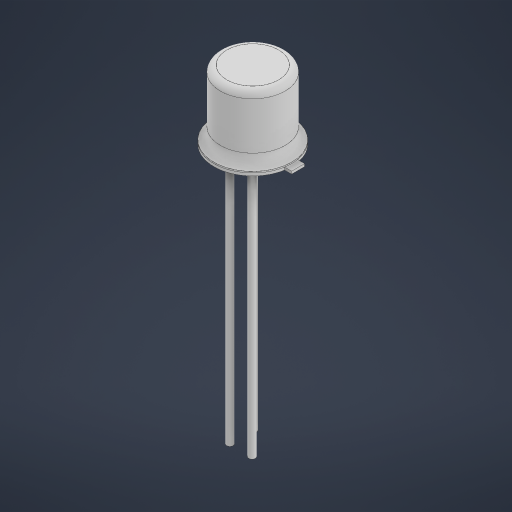
# Autodesk Inventor part: Part4
Saved by Autodesk Inventor 2024 (Build 280153000, 153)
## iProperties
Created: 2023-12-19
Part Number: Part4
Material: Generic
Document SubType Name: Sheet Metal
Designer: Shado
Density: 1 g/cm^3
Sheet Metal Rule: Default
Appearance: Default
Author: Shado
Autodesk Inventor part; units mm, degrees
ref_plane "YZ Plane" through (0, 0, 0) normal (1, 0, 0) x (0, 1, 0)
ref_plane "XZ Plane" through (0, 0, 0) normal (0, 1, 0) x (-1, 0, 0)
ref_plane "XY Plane" through (0, 0, 0) normal (0, 0, 1) x (1, 0, 0)
sketch "Sketch1" plane through (0, 0, 0) normal (0, 1, 0) x (-1, 0, 0)
  arc A0 (-2.958, -0.5) -> (-2.958, 0.5) centre (0, 0) ccw
  line L0 (-3.5, 0) -> (-3.5, -0.5)
  line L1 (-3.5, -0.5) -> (-3, -0.5)
  line L2 (-3, -0.5) -> (-2.958, -0.5)
  line L3 (-3.5, 0) -> (-3.5, 0.5)
  line L4 (-3.5, 0.5) -> (-2.958, 0.5)
  dimension "d0" = 6
  dimension "d1" = 0.5
  dimension "d2" = 0.5
  dimension "d3" = 0.5
  constraints: 10 end point, 2 point on circle, 1 centre point, 1 coincident, 1 horizontal, 1 perpendicular, 1 vertical
  measures "d0" diameter of A0
  measures "d1" distance of L1.end L0.end
  measures "d2" distance of L0.end L0.start
  measures "d3" distance of L0.start L3.end
extrude "Extrusion1" add sketch "Sketch1" along normal blind 0.2
sketch "Sketch2" plane through (0, 0.2, 0) normal (0, 1, 0) x (1, 0, 0)
  circle A0 centre (0, 0) radius 2.9999
  constraints: 1 centre point, 1 coincident
extrude "Extrusion2" add sketch "Sketch2" along normal blind 0.1
sketch "Sketch3" plane through (0, 0.3, 0) normal (0, 1, 0) x (1, 0, 0)
  circle A0 centre (0, 0) radius 2.5
  dimension "d8" = 5
  constraints: 1 centre point, 1 coincident
  measures "d8" diameter of A0
extrude "Extrusion3" add sketch "Sketch3" along normal blind 5
fillet "Fillet1" radius 0.5 1 edges at (-2.5, 5.3, 0)
fillet "Fillet2" radius 1 1 edges at (-2.5, 0.3, 0)
sketch "Sketch4" plane through (0, 0, 0) normal (0, -1, 0) x (1, 0, 0)
  circle A0 centre (0, 0) radius 1.25
  circle A1 centre (0.8555, -0.9113) radius 0.25
  circle A2 centre (0.8555, 0.9113) radius 0.25
  circle A3 centre (-0.8555, -0.9113) radius 0.25
  circle A4 centre (-0.8555, 0.9113) radius 0.25
  dimension "d13" = 2.5
  dimension "d14" = 0.5
  dimension "d16" = 0.5
  dimension "d17" = 0.5
  dimension "d18" = 0.5
  constraints: 5 centre point, 4 point on circle, 1 coincident
  measures "d13" diameter of A0
  measures "d14" diameter of A1
  measures "d16" diameter of A2
  measures "d17" diameter of A3
  measures "d18" diameter of A4
extrude "Extrusion4" add sketch "Sketch4" along normal blind 20 contours A2 A0 | A0 A2 | A4 A0 | A0 A4 | A3 A0 | A0 A3
equation "\"BendRadius\" = Thickness"
equation "\"BendReliefWidth\" = Thickness"
equation "\"BendReliefDepth\" = 0.5 * Thickness"
equation "\"CornerReliefSize\" = 4 * Thickness"
equation "\"MinimumRemnant\" = 2 * Thickness"
equation "\"TransitionRadius\" = BendRadius"
equation "\"JacobiRadiusSize\" = BendRadius"
equation "\"GapSize\" = Thickness"
equation "\"Thickness\" = 3.048"
body "Solid1"
